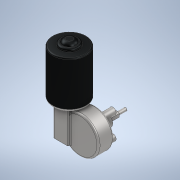
# Autodesk Inventor part: motor
Saved by Autodesk Inventor 2021 (Build 250183000, 183)
## iProperties
Created: 2020-10-28
Part Number: motor
Material: Generic
Document SubType Name: Modeling
Designer: Mateusz
Density: 1 g/cm^3
Appearance: Default
Author: Mateusz
Autodesk Inventor part; units mm, degrees
ref_plane "YZ Plane" through (0, 0, 0) normal (1, 0, 0) x (0, 1, 0)
ref_plane "XZ Plane" through (0, 0, 0) normal (0, 1, 0) x (-1, 0, 0)
ref_plane "XY Plane" through (0, 0, 0) normal (0, 0, 1) x (1, 0, 0)
sketch "Sketch1" plane through (0, 0, 0) normal (0, 1, 0) x (-1, 0, 0)
  circle A0 centre (0, 0) radius 31
  dimension "d0" = 62
  constraints: 1 centre point, 1 coincident
  measures "d0" diameter of A0
extrude "Extrusion1" add sketch "Sketch1" along normal blind 87
sketch "Sketch2" plane through (0, 0, 0) normal (0, 1, 0) x (-1, 0, 0)
  line L0 (0, 0) -> (0, -36.5)
  line L1 (0, -36.5) -> (-33, -36.5)
  line L2 (-33, -36.5) -> (-33, 13.5)
  line L3 (-33, 13.5) -> (0, 13.5)
  dimension "d3" = 36.5
  dimension "d4" = 33
  dimension "d15" = 50
  constraints: 8 end point, 2 perpendicular, 2 vertical
  measures "d3" distance of L0.start L0.end
  measures "d4" distance of L0.end L1.end
  measures "d15" distance of L1.end L2.end
sketch "Sketch3" plane through (0, 0, 0) normal (0, 0, 1) x (1, 0, 0)
  line L0 (0, 0) -> (33, 0) projected
  circle A0 centre (33, -35.5) radius 34.5
  circle A1 centre (8.5, -35.5) radius 3
  circle A2 centre (45.25, -56.7176) radius 3
  circle A3 centre (45.25, -14.2824) radius 3
  dimension "d13" = 360
  constraints: 4 centre point, 1 coincident, 7 other
extrude "Extrusion2" add sketch "Sketch3" along normal up to surface (13.5 mm away) contours A0 | A1 | A2 | A3
extrude "Extrusion3" add sketch "Sketch3" against normal blind 15 contours A0 | A1 | A2 | A3
sketch "Sketch4" plane through (33, -35.5, -15) normal (0, 0, -1) x (-1, 0, 0)
  point P0 (33, 35.5)
extrude "Extrusion4" add sketch "Sketch3" against normal blind 30 contours A1 | A2 | A3
sketch "Sketch5" plane through (33, -35.5, -15) normal (0, 0, -1) x (-1, 0, 0)
  circle A0 centre (-12.25, 21.2176) radius 3 projected
  circle A1 centre (-12.25, 21.2176) radius 6
  circle A2 centre (24.5, 0) radius 3 projected
  circle A3 centre (24.5, 0) radius 6
  circle A4 centre (-12.25, -21.2176) radius 3 projected
  circle A5 centre (-12.25, -21.2176) radius 6
  point P0 (33, 35.5)
  dimension "d22" = 12
  dimension "d23" = 12
  dimension "d24" = 12
  constraints: 3 centre point, 3 coincident
  measures "d22" diameter of A1
  measures "d23" diameter of A3
  measures "d24" diameter of A5
extrude "Extrusion5" add sketch "Sketch5" along normal blind 20.5
sketch "Sketch6" plane through (0, 0, 0) normal (0, -1, 0) x (1, 0, 0)
  line L0 (0, 0) -> (-10, 0)
  line L1 (-10, 0) -> (-10, 10.9901)
  line L2 (0, 0) -> (10, 0)
  line L3 (10, 0) -> (10, 10.9901)
  line L4 (10, 13.9901) -> (10, 10.9901)
  line L5 (10, 10.9901) -> (15, 10.9901)
  line L6 (15, 10.9901) -> (15, 17.1966)
  line L7 (-12.9999, 16.98) -> (-12.9999, 10.9901)
  line L8 (-12.9999, 10.9901) -> (-10, 10.9901)
  arc A0 (-12.9999, 11.2572) -> (13.2265, 10.9901) centre (0, 0) ccw
  line L9 (15, 17.1966) -> (-12.9999, 17.1966)
  line L10 (-12.9999, 17.1966) -> (-12.9999, 16.98)
  circle A1 centre (0, 0) radius 10
  dimension "d27" = 10
  dimension "d28" = 10
  dimension "d29" = 3
  dimension "d30" = 5
  constraints: 22 end point, 5 perpendicular, 5 point on line, 2 coincident, 2 horizontal, 2 point on circle, 1 centre point, 1 parallel, 3 other
  measures "d27" distance of L0.start L0.end
  measures "d28" distance of L0.start L2.end
  measures "d29" distance of L3.end L4.start
  measures "d30" distance of L3.end L5.end
extrude "Extrusion6" add sketch "Sketch6" along normal blind 5 contours A1 L3 L5 A0 L7 L8 L1
extrude "Extrusion7" add sketch "Sketch6" along normal blind 60 contours L2 A1 L0 | L0 A1 L2 | L1 L8 L7 L10 L9 L6 L5 L3 A1
sketch "Sketch7" plane through (33, -35.5, -15) normal (0, 0, -1) x (-1, 0, 0)
  circle A0 centre (0, 0) radius 11
  point P0 (33, 35.5)
  dimension "d48" = 22
  constraints: 1 centre point
  measures "d48" diameter of A0
extrude "Extrusion8" add sketch "Sketch7" along normal blind 21.5
sketch "Sketch8" plane through (0, 87, 0) normal (0, 1, 0) x (1, 0, 0)
  circle A0 centre (0, 0) radius 17.1966
  constraints: 1 centre point, 1 coincident
extrude "Extrusion9" add sketch "Sketch8" along normal blind 5
sketch "Sketch9" plane through (0, 92, 0) normal (0, 1, 0) x (1, 0, 0)
  circle A0 centre (0, 0) radius 12.4501
  constraints: 1 centre point, 1 coincident
extrude "Extrusion10" add sketch "Sketch9" along normal blind 5
fillet "Fillet1" radius 3 1 edges at (-17.1966, 92, 0)
fillet "Fillet1" radius 7 1 edges at (-12.4501, 97, 0)
fillet "Fillet2" radius 2 1 edges at (31, 87, 0)
fillet "Fillet3" radius 2 4 edges at (15, -30, 17.1966) (15, -33.0339, 13.5) (-12.9999, -30, 17.1966) (-12.9999, -32.5, 10.9901)
fillet "Fillet4" radius 2 1 edges at (-0.5016, 0, -17.1893)
sketch "Sketch10" plane through (33, -35.5, -36.5) normal (0, 0, -1) x (-1, 0, 0)
  circle A0 centre (0, 0) radius 5
  point P0 (33, 35.5)
  dimension "d49" = 10
  constraints: 1 centre point
  measures "d49" diameter of A0
extrude "Extrusion11" add sketch "Sketch10" along normal blind 19
sketch "Sketch11" plane through (33, -35.5, -55.5) normal (0, 0, -1) x (-1, 0, 0)
  line L0 (0, 0) -> (4, 0)
  line L1 (4, 0) -> (-4, 0)
  line L2 (-4, 0) -> (-4, -3)
  circle A0 centre (0, 0) radius 5 projected
  line L3 (-4, 0) -> (-4, 3)
  line L4 (4, 0) -> (4, -3)
  line L5 (4, 0) -> (4, 3)
  point P0 (33, 35.5)
  dimension "d52" = 4
  dimension "d53" = 8
  constraints: 12 end point, 4 point on circle, 3 point on line, 1 horizontal, 1 parallel, 1 perpendicular
  measures "d52" distance of L0.start L0.end
  measures "d53" distance of L0.end L1.end
extrude "Extrusion12" cut sketch "Sketch11" against normal blind 15.5 contours L5 A0 L4 | L2 A0 L3
sketch "Sketch12" plane through (33, -35.5, -55.5) normal (0, 0, -1) x (-1, 0, 0)
  circle A0 centre (0, 0) radius 5 projected
  circle A1 centre (0, 0) radius 3
  point P0 (33, 35.5)
  dimension "d56" = 6
  constraints: 1 centre point, 1 coincident
  measures "d56" diameter of A1
extrude "Extrusion13" add sketch "Sketch12" along normal blind 15.5 contours A1
fillet "Fillet5" radius 5 1 edges at (31, 0, 0)
sketch "Sketch13" plane through (33, -35.5, -15) normal (0, 0, -1) x (-1, 0, 0)
  circle A0 centre (0, 0) radius 3 projected
  circle A1 centre (0, 0) radius 25
  circle A2 centre (0, 0) radius 24
  line L0 (0, -24) -> (0, -25)
  circle A3 centre (0, -24.5) radius 2
  circle A4 centre (-12.25, -21.2176) radius 3 projected
  circle A5 centre (0, 0) radius 5 projected
  circle A6 centre (-21.2176, -12.2501) radius 2
  circle A7 centre (21.2177, -12.2499) radius 2
  circle A8 centre (21.2176, 12.25) radius 2
  circle A9 centre (-0.0001, 24.5) radius 2
  circle A10 centre (-21.2176, 12.25) radius 2
  point P0 (33, 35.5)
  point P1 (-1.9151, -23.9235)
  point P2 (-9.38, -22.0911)
  point P3 (-14.4415, -19.1688)
  point P4 (-19.7607, -13.6204)
  point P5 (-21.6758, -10.3033)
  point P6 (-21.6759, 10.3032)
  point P7 (-19.7608, 13.6203)
  point P8 (-1.9152, 23.9235)
  point P9 (1.915, 23.9235)
  point P10 (19.7608, 13.6203)
  point P11 (21.6759, 10.3032)
  point P12 (21.6759, -10.3031)
  point P13 (19.7609, -13.6201)
  point P14 (1.9151, -23.9235)
  point P15 (-1.9547, -24.9235)
  point P16 (1.9547, -24.9235)
  point P17 (20.6071, -14.1544)
  point P18 (22.5617, -10.7688)
  point P19 (22.5617, 10.769)
  point P20 (20.607, 14.1545)
  point P21 (1.9545, 24.9235)
  point P22 (-1.9548, 24.9235)
  point P23 (-20.607, 14.1545)
  point P24 (-22.5617, 10.769)
  point P25 (-22.5616, -10.7691)
  point P26 (-20.607, -14.1546)
  dimension "d60" = 50
  dimension "d61" = 48
  dimension "d62" = 4
  dimension "d65" = 4
  dimension "d68" = 360
  constraints: 6 centre point, 2 coincident, 2 end point, 1 midpoint, 1 vertical, 19 other
  measures "d62" diameter of A3
  measures "d65" diameter of A6
extrude "Extrusion14" add sketch "Sketch13" along normal blind 3 contours A0 | A1 A7 A2 A8 | A8 A2 A1 | A1 A8 | A7 A1 | A1 A7 A2 | A8 A2 A9 A1 | A8 A2 | A1 A3 A2 A7 | A2 A7 | A9 A2 A1 | A1 A9 | A3 A1 | A1 L0 A2 A3 | A9 A2 A10 A1 | A9 A2 | A1 A3 A2 L0 | A1 A4 A2 A3 | A2 A3 | A10 A2 A1 | A1 A10 | A1 A4 A2 | A10 A2 A6 A1 | A10 A2 | A1 A6 A2 A4 | A2 A4 | A6 A2 A1 | A1 A6 | A6 A2 | A5
sketch "Sketch14" plane through (0, 0, -15) normal (0, 0, -1) x (-1, 0, 0)
  circle A0 centre (-45.25, -14.2824) radius 3 projected
  circle A1 centre (-33, -35.5) radius 3 projected
  circle A2 centre (-8.5, -35.5) radius 3 projected
  line L0 (-8.5, -35.5) -> (-33, -35.5)
  circle A3 centre (-33, -35.5) radius 5 projected
  circle A4 centre (-45.25, -56.7176) radius 3 projected
  line L1 (-45.25, -56.7176) -> (-44.384, -57.2176)
  line L2 (-44.384, -57.2176) -> (-37.6112, -45.4868)
  circle A5 centre (-33, -35.5) radius 11 projected
  line L3 (-45.25, -56.7176) -> (-46.116, -56.2176)
  line L4 (-46.116, -56.2176) -> (-39.3433, -44.4868)
  line L5 (-8.5, -35.5) -> (-8.5, -36.5)
  line L6 (-8.5, -36.5) -> (-22.0455, -36.5)
  line L7 (-8.5, -35.5) -> (-8.5, -34.5)
  line L8 (-8.5, -34.5) -> (-22.0455, -34.5)
  line L9 (-45.25, -14.2824) -> (-46.116, -14.7824)
  line L10 (-46.116, -14.7824) -> (-39.3433, -26.5132)
  line L11 (-45.25, -14.2824) -> (-44.384, -13.7824)
  line L12 (-44.384, -13.7824) -> (-37.6112, -25.5132)
  circle A6 centre (-45.25, -14.2824) radius 6 projected
  circle A7 centre (-33, -35.5) radius 11 projected
  circle A8 centre (-8.5, -35.5) radius 6 projected
  circle A9 centre (-45.25, -56.7176) radius 6 projected
  point P0 (0, 0)
  point P1 (-14.4161, -36.5)
  point P2 (-14.4161, -34.5)
  point P3 (-43.158, -51.0941)
  point P4 (-41.4259, -52.0941)
  point P5 (-41.4259, -18.9059)
  point P6 (-43.158, -19.9059)
  dimension "d72" = 1
  dimension "d73" = 1
  dimension "d74" = 1
  dimension "d75" = 1
  dimension "d76" = 1
  dimension "d77" = 1
  constraints: 26 end point, 6 perpendicular, 5 point on circle, 3 point on line
  measures "d72" distance of L1.start L1.end
  measures "d73" distance of L1.start L3.end
  measures "d74" distance of L0.start L5.end
  measures "d75" distance of L0.start L7.end
  measures "d76" distance of L9.start L9.end
  measures "d77" distance of L9.start L11.end
extrude "Extrusion15" add sketch "Sketch14" along normal blind 12 contours A6 L12 A5 L10 | A5 L2 A9 L4 | L8 A8 L0 A5 | L0 A8 L6 A5
fillet "Fillet6" radius 3 1 edges at (-1.5, -35.5, -15)
fillet "Fillet7" radius 3 3 edges at (15.5941, -5.7127, 14.0662) (50.8585, -5.9818, 13.5) (46.2712, -67.3453, 13.5)
body "Solid1"
